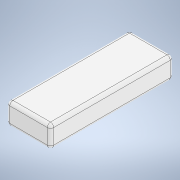
# Autodesk Inventor part: battery
Saved by Autodesk Inventor 2021 (Build 250183000, 183)
## iProperties
Created: 2022-05-14
Part Number: battery
Material: Generic
Document SubType Name: Modeling
Designer: ermoz
Density: 1 g/cm^3
Appearance: Default
Author: ermoz
Autodesk Inventor part; units mm, degrees
ref_plane "YZ Plane" through (0, 0, 0) normal (1, 0, 0) x (0, 1, 0)
ref_plane "XZ Plane" through (0, 0, 0) normal (0, 1, 0) x (-1, 0, 0)
ref_plane "XY Plane" through (0, 0, 0) normal (0, 0, 1) x (1, 0, 0)
sketch "Sketch1" plane through (0, 0, 0) normal (0, 1, 0) x (-1, 0, 0)
  line L0 (0, 0) -> (27.5, 0)
  line L1 (27.5, 0) -> (27.5, 77)
  line L2 (27.5, 77) -> (0, 77)
  line L3 (0, 77) -> (0, 0)
  dimension "d0" = 77
  dimension "d1" = 27.5
  constraints: 8 end point, 2 parallel, 1 horizontal, 1 perpendicular
  measures "d0" distance of L0.end L1.end
  measures "d1" distance between parallel lines of L3 L1
extrude "Extrusion1" add sketch "Sketch1" along normal blind 13.5
fillet "Fillet1" radius 2 12 edges at (0, 13.5, 38.5) (0, 0, 38.5) (-27.5, 13.5, 38.5) (-27.5, 0, 38.5) (-13.75, 13.5, 0) (-27.5, 6.75, 0) (-13.75, 0, 0) (0, 6.75, 0) (0, 6.75, 77) (-13.75, 0, 77) (-13.75, 13.5, 77) (-27.5, 6.75, 77)
body "Solid1"
